test cut HDPE on small machine or burrs_v1 (Autodesk Fusion 360 design; units mm, degrees)
Autodesk Fusion 360 part; units mm, degrees
sketch "lines" plane through (0, 0, 0) normal (0, 0, 1) x (1, 0, 0)
  circle A0 centre (-302, 114) radius 1.05
  circle A1 centre (-154, 222) radius 1.05
  circle A2 centre (-302, 222) radius 1.05
  line L0 (2, 11.8017) -> (8, 11.8017)
  line L1 (8, 11.8017) -> (8, 2)
  line L2 (8, 2) -> (2, 2)
  line L3 (2, 2) -> (2, 11.8017)
  line L4 (19.2, 2) -> (13.2, 2)
  line L5 (13.2, 2) -> (13.2, 11.8017)
  line L6 (19.2, 11.8017) -> (19.2, 2)
  line L7 (13.2, 11.8017) -> (19.2, 11.8017)
  line L8 (1.75, 0) -> (22.5, 0)
  point P0 (11.2, 0)
  dimension "d488" = 6
  dimension "d491" = 11.2
  dimension "d492" = 0
  dimension "d495" = 2
  dimension "d496" = 2
  constraint horizontal L0
  constraint vertical L1
  constraint horizontal L2
  constraint vertical L3
  measures "d488" distance of L0.start L0.end
  measures "d495" distance of origin L3
  measures "d496" distance of L2 L8
pattern_linear "bottom length repeat holes" [no effect]
extrude "Extrude21" add sketch "lines" along normal blind 3.175 contours L0 L1 L2 L3 | L4 L5 L6 L7 makes body 1 at (17.2, 5.2672, 0) makes body 2 at (6, 8.5345, 0)
equation "fingerWidth = 10 mm"
equation "length = 160 mm"
equation "thickness = 3.175 mm"
equation "height = 50 mm"
equation "d21 = lengthCutsBottom"
equation "d23 = -2 * fingerWidth"
equation "toolDiameter = 1.401 mm"
equation "boneCornerToCenter = toolDiameter / 2 / sqrt(2) - 0 * kerf" comment "Best: 2.001 -2*kerf, 0.1;;;Best: 2.001 no kerf and 0.1   OLD+6 kerf at 2.001 Diam and .1 mm"
equation "tempLengthPiecesBottom = ceil(( ( floor(( length - 2 * thickness ) / fingerWidth) - 2 ) - ( ( floor(( length - 2 * thickness ) / fingerWidth) - 2 ) % 2 - 1 ) ))"
equation "lengthCutsBottom = ceil(tempLengthPiecesBottom / 2)"
equation "lengthShoulder = ( length - fingerWidth * tempLengthPiecesBottom ) / 2 - kerf"
equation "depth = 120 mm"
equation "tempDepthPiecesBottom = ceil(( ( floor(( depth - 2 * thickness ) / fingerWidth) - 2 ) - ( ( floor(( depth - 2 * thickness ) / fingerWidth) - 2 ) % 2 - 1 ) ))"
equation "depthCutsSideBottom = ceil(tempDepthPiecesBottom / 2)"
equation "depthShoulder = ( depth - fingerWidth * tempDepthPiecesBottom ) / 2 - kerf"
equation "tempHeightPiecesSide = ceil(( ( floor(( height - 2 * thickness ) / fingerWidth) - 2 ) - ( ( floor(( height - 2 * thickness ) / fingerWidth) - 2 ) % 2 - 1 ) ))"
equation "heightCutsSide = ceil(tempHeightPiecesSide / 2)"
equation "heightSholder = ( height - fingerWidth * tempHeightPiecesSide ) / 2 - kerf"
equation "kerf = -0.093 mm"
equation "holeWidth = fingerWidth + 2 * kerf"
equation "lengthShoulderHole = lengthShoulder + 2 * kerf"
equation "depthShouderHole = depthShoulder + 2 * kerf"
equation "heightShoulderHole = heightSholder + 2 * kerf"
equation "assembleScrewDiam = 2.1 mm"
equation "assembleScrewDistance = 6 mm"
equation "assembleAvoidCollisionDistance = 1 mm"
equation "coolingHoleDistance = 8 mm"
equation "boneCornerToCenterPack = -3 * kerf"
equation "boneCornerToCenterSide = boneCornerToCenter - boneCornerToCenterPack"
